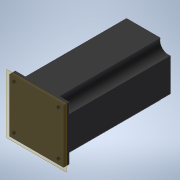
# Autodesk Inventor part: nema23
Saved by Autodesk Inventor 2020 (Build 240168000, 168)
## iProperties
Created: 2021-09-05
Part Number: nema23
Material: Generic
Document SubType Name: Modeling
Designer: super
Density: 1 g/cm^3
Appearance: Default
Author: super
Autodesk Inventor part; units mm, degrees
ref_plane "YZ Plane" through (0, 0, 0) normal (1, 0, 0) x (0, 1, 0)
ref_plane "XZ Plane" through (0, 0, 0) normal (0, 1, 0) x (-1, 0, 0)
sketch "Sketch1" plane through (0, 0, 0) normal (0, 0, 1) x (1, 0, 0)
  line L0 (0, 0) -> (57, 0)
  line L1 (57, 0) -> (57, 57)
  line L2 (57, 57) -> (0, 57)
  line L3 (0, 57) -> (0, 0)
  circle A0 centre (5, 5) radius 2.5
  circle A1 centre (52, 5) radius 2.5
  circle A2 centre (5, 52) radius 2.5
  circle A3 centre (52, 52) radius 2.5
  dimension "d0" = 57
  dimension "d1" = 57
  dimension "d2" = 5
  dimension "d3" = 5
  dimension "d4" = 5
  constraints: 8 end point, 4 centre point, 2 parallel, 1 horizontal, 1 perpendicular
  measures "d0" distance of L2.end L1.end
  measures "d1" distance of L1.end L0.end
  measures "d2" diameter of A0
  measures "d3" horizontal distance of L0.start A0.centre
  measures "d4" horizontal distance of L0.start A0.centre
extrude "Extrusion1" add sketch "Sketch1" against normal blind 113
sketch "Sketch2" plane through (0, 0, -113) normal (0, 0, -1) x (-1, 0, 0)
  line L0 (0, 57) -> (-57, 57) projected
  line L1 (-28.5, 57) -> (-28.5, 0)
  line L2 (-57, 0) -> (0, 0) projected
  line L3 (-57, 57) -> (-57, 0) projected
  line L4 (-57, 28.5) -> (0, 28.5)
  line L5 (0, 0) -> (0, 57) projected
  arc A0 (-46.3441, 0) -> (-57, 10.9524) centre (-54.7847, 2.4478) ccw
  line L6 (-57, 10.9524) -> (-57, 0)
  line L7 (0, 0) -> (-57, 0)
  line L8 (0, 57) -> (0, 0)
  arc A1 (0, 10.9524) -> (-10.6559, 0) centre (-2.2153, 2.4478) ccw
  line L9 (-57, 57) -> (0, 57)
  arc A2 (-57, 46.0476) -> (-46.3441, 57) centre (-54.7847, 54.5522) ccw
  line L10 (-57, 46.0476) -> (-57, 57)
  arc A3 (-10.6559, 57) -> (0, 46.0476) centre (-2.2153, 54.5522) ccw
  line L11 (0, 57) -> (-57, 57)
  point P0 (0, 10.9524)
  point P1 (-10.6559, 0)
  point P2 (-10.6559, 57)
  point P3 (0, 46.0476)
  point P4 (-46.3441, 57)
  constraints: 16 end point, 15 symmetric about line, 8 point on circle, 6 point on line, 4 centre point, 4 midpoint, 1 vertical, 3 other
extrude "Extrusion2" cut sketch "Sketch2" against normal blind 107 contours L5 A3 L0 | A2 L3 L0 | L5 L2 A1 | L2 L3 A0
body "Solid1"
